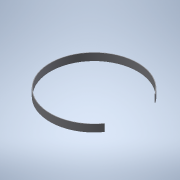
# Autodesk Inventor part: Floor Banding
Saved by Autodesk Inventor 2021 (Build 250183000, 183)
## iProperties
Created: 2020-07-30
Part Number: Floor Banding
Material: Generic
Document SubType Name: Modeling
Designer: Dan Wikman
Density: 1 g/cm^3
Appearance: Default
Author: Dan Wikman
Autodesk Inventor part; units mm, degrees
ref_plane "YZ Plane" through (0, 0, 0) normal (1, 0, 0) x (0, 1, 0)
ref_plane "XZ Plane" through (0, 0, 0) normal (0, 1, 0) x (-1, 0, 0)
ref_plane "XY Plane" through (0, 0, 0) normal (0, 0, 1) x (1, 0, 0)
sketch "Sketch1" plane through (0, 0, 0) normal (0, 1, 0) x (-1, 0, 0)
  arc A0 (-244.8181, -173.39) -> (-244.9625, 173.1859) centre (0, 0) ccw
  line L0 (290, 3.75) -> (260, 3.75)
  line L1 (260, -3.75) -> (290, -3.75)
  arc A1 (291.75, 2) -> (290, 3.75) centre (290, 2) ccw
  arc A2 (290, -3.75) -> (291.75, -2) centre (290, -2) ccw
  arc A3 (258.25, -2) -> (260, -3.75) centre (260, -2) ccw
  arc A4 (260, 3.75) -> (258.25, 2) centre (260, 2) ccw
  line L2 (258.25, 2) -> (258.25, -2)
  line L3 (291.75, -2) -> (291.75, 2)
  line L4 (306.241, 0) -> (300, 0)
  line L5 (300, 0) -> (281.7438, 0)
  line L6 (86.0485, 276.9652) -> (76.778, 248.4335)
  arc A5 (88.2536, 278.0888) -> (86.0485, 276.9652) centre (87.7128, 276.4244) ccw
  line L7 (92.0578, 276.8527) -> (88.2536, 278.0888)
  line L8 (83.9109, 246.1159) -> (93.1814, 274.6476)
  arc A6 (93.1814, 274.6476) -> (92.0578, 276.8527) centre (91.517, 275.1884) ccw
  arc A7 (76.778, 248.4335) -> (77.9015, 246.2284) centre (78.4423, 247.8927) ccw
  line L9 (77.9015, 246.2284) -> (81.7058, 244.9923)
  arc A8 (81.7058, 244.9923) -> (83.9109, 246.1159) centre (82.2465, 246.6567) ccw
  line L10 (-236.8191, 167.4239) -> (-212.5486, 149.7904)
  arc A9 (-237.2063, 169.8683) -> (-236.8191, 167.4239) centre (-235.7905, 168.8397) ccw
  line L11 (-234.8551, 173.1044) -> (-237.2063, 169.8683)
  line L12 (-208.1402, 155.858) -> (-232.4107, 173.4915)
  arc A10 (-232.4107, 173.4915) -> (-234.8551, 173.1044) centre (-233.4394, 172.0758) ccw
  arc A11 (-212.5486, 149.7904) -> (-210.1042, 150.1775) centre (-211.52, 151.2061) ccw
  line L13 (-210.1042, 150.1775) -> (-207.7531, 153.4136)
  arc A12 (-207.7531, 153.4136) -> (-208.1402, 155.858) centre (-209.1688, 154.4422) ccw
  line L14 (-232.4107, -173.4915) -> (-208.1402, -155.858)
  arc A13 (-234.8551, -173.1044) -> (-232.4107, -173.4915) centre (-233.4394, -172.0758) ccw
  line L15 (-237.2063, -169.8683) -> (-234.8551, -173.1044)
  line L16 (-212.5486, -149.7904) -> (-236.8191, -167.4239)
  arc A14 (-236.8191, -167.4239) -> (-237.2063, -169.8683) centre (-235.7905, -168.8397) ccw
  arc A15 (-208.1402, -155.858) -> (-207.7531, -153.4136) centre (-209.1688, -154.4422) ccw
  line L17 (-207.7531, -153.4136) -> (-210.1042, -150.1775)
  arc A16 (-210.1042, -150.1775) -> (-212.5486, -149.7904) centre (-211.52, -151.2061) ccw
  line L18 (93.1814, -274.6476) -> (83.9109, -246.1159)
  arc A17 (92.0578, -276.8527) -> (93.1814, -274.6476) centre (91.517, -275.1884) ccw
  line L19 (88.2536, -278.0888) -> (92.0578, -276.8527)
  line L20 (76.778, -248.4335) -> (86.0485, -276.9652)
  arc A18 (86.0485, -276.9652) -> (88.2536, -278.0888) centre (87.7128, -276.4244) ccw
  arc A19 (83.9109, -246.1159) -> (81.7058, -244.9923) centre (82.2465, -246.6567) ccw
  line L21 (81.7058, -244.9923) -> (77.9015, -246.2284)
  arc A20 (77.9015, -246.2284) -> (76.778, -248.4335) centre (78.4423, -247.8927) ccw
  arc A21 (-248.0544, -175.7413) -> (-248.1989, 175.5373) centre (0, 0) ccw
  line L22 (-244.8181, -173.39) -> (-248.0544, -175.7413)
  line L23 (-244.9625, 173.1859) -> (-248.1989, 175.5373)
  point P0 (87.0636, 267.9543)
  point P1 (-227.9355, 165.6049)
  point P2 (-227.9355, -165.6049)
  point P3 (87.0636, -267.9543)
  dimension "d3" = 7.5
  dimension "d6" = 30
  dimension "d7" = 3.5
  dimension "d8" = 3.5
  dimension "d26" = 8.25
  dimension "d27" = 33.5
  dimension "d28" = 7.5
  dimension "d43" = 4
  dimension "d46" = 0.125
  dimension "d47" = 0.125
  constraints: 48 end point, 45 point on circle, 22 centre point, 4 tangent, 3 horizontal, 1 coincident, 1 parallel, 1 perpendicular, 44 other
  measures "d3" distance between parallel lines of L1 L0
  measures "d6" distance of L1.start L1.end
  measures "d7" diameter of A1
  measures "d8" diameter of A2
  measures "d26" distance from line of L4.end L3
  measures "d27" distance between parallel lines of L2 L3
  measures "d28" diameter of L1 L5
  measures "d43" radial gap between concentric circles of A0 A21
  measures "d46" distance between parallel lines of L23 L10
  measures "d47" distance between parallel lines of L16 L22
extrude "Extrusion3" add sketch "Sketch1" along normal blind 50 contours A0 L4 A21 L22 | A0 L23 A21 L4
body "Solid2"
